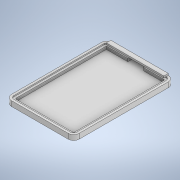
# Autodesk Inventor part: piholder-v1
Saved by Autodesk Inventor 2022 (Build 260153000, 153)
## iProperties
Created: 2021-07-08
Part Number: piholder-v1
Material: Generic
Document SubType Name: Modeling
Designer: dncob
Density: 1 g/cm^3
Appearance: Default
Author: dncob
Autodesk Inventor part; units mm, degrees
ref_plane "YZ Plane" through (0, 0, 0) normal (1, 0, 0) x (0, 1, 0)
ref_plane "XZ Plane" through (0, 0, 0) normal (0, 1, 0) x (-1, 0, 0)
ref_plane "XY Plane" through (0, 0, 0) normal (0, 0, 1) x (1, 0, 0)
sketch "Sketch1" plane through (0, 0, 0) normal (0, 1, 0) x (-1, 0, 0)
  line L0 (-25, 42.5) -> (25, 42.5)
  line L1 (28, 39.5) -> (28, -40.5)
  line L2 (26, -42.5) -> (-25, -42.5)
  line L3 (-28, -39.5) -> (-28, 39.5)
  line L4 (-28, 42.5) -> (28, -42.5) construction
  line L5 (28, 42.5) -> (-28, -42.5) construction
  arc A0 (26, -42.5) -> (28, -40.5) centre (26, -40.5) ccw
  arc A1 (-28, -39.5) -> (-25, -42.5) centre (-25, -39.5) ccw
  arc A2 (-25, 42.5) -> (-28, 39.5) centre (-25, 39.5) ccw
  arc A3 (28, 39.5) -> (25, 42.5) centre (25, 39.5) ccw
  line L6 (30, -40.5) -> (30, 39.5)
  arc A4 (30, 39.5) -> (25, 44.5) centre (25, 39.5) ccw
  line L7 (25, 44.5) -> (-25, 44.5)
  arc A5 (-25, 44.5) -> (-30, 39.5) centre (-25, 39.5) ccw
  line L8 (-30, 39.5) -> (-30, -39.5)
  arc A6 (-30, -39.5) -> (-25, -44.5) centre (-25, -39.5) ccw
  line L9 (-25, -44.5) -> (26, -44.5)
  arc A7 (26, -44.5) -> (30, -40.5) centre (26, -40.5) ccw
  point P0 (0, 0)
  dimension "d0" = 56
  dimension "d1" = 85
  dimension "d2" = 2
  dimension "d3" = 3
  dimension "d4" = 2
  constraints: 20 end point, 16 point on circle, 8 centre point, 8 point on line, 8 tangent, 4 parallel, 2 equal radius, 2 midpoint, 2 perpendicular, 1 horizontal, 7 other
  measures "d0" distance of L4.end L5.end
  measures "d1" distance of L5.start L4.end
  measures "d2" radius of A0
  measures "d3" radius of A1
  measures "d4" distance between parallel lines of L1 L6
extrude "Extrusion1" add sketch "Sketch1" along normal blind 1
sketch "Sketch2" plane through (0, 0, 0) normal (0, -1, 0) x (1, 0, 0)
  arc A0 (-25, 44.5) -> (-30, 39.5) centre (-25, 39.5) ccw projected
  line L0 (-25, 44.5) -> (25, 44.5) projected
  arc A1 (30, 39.5) -> (25, 44.5) centre (25, 39.5) ccw projected
  line L1 (30, 39.5) -> (30, -39.5) projected
  arc A2 (25, -44.5) -> (30, -39.5) centre (25, -39.5) ccw projected
  line L2 (25, -44.5) -> (-26, -44.5) projected
  arc A3 (-30, -40.5) -> (-26, -44.5) centre (-26, -40.5) ccw projected
  line L3 (-30, -40.5) -> (-30, 39.5) projected
  line L4 (-26, -44.5) -> (25, -44.5)
  line L5 (30, -39.5) -> (30, 39.5)
  line L6 (25, 44.5) -> (-25, 44.5)
  line L7 (-30, 39.5) -> (-30, -40.5)
  line L8 (-30, -44.5) -> (30, 44.5) construction
  line L9 (30, -44.5) -> (-30, 44.5) construction
  arc A4 (-25, 44.5) -> (-30, 39.5) centre (-25, 39.5) ccw
  arc A5 (30, 39.5) -> (25, 44.5) centre (25, 39.5) ccw
  arc A6 (25, -42.5) -> (28, -39.5) centre (25, -39.5) ccw projected
  arc A7 (25, -44.5) -> (30, -39.5) centre (25, -39.5) ccw
  arc A8 (-30, -40.5) -> (-26, -44.5) centre (-26, -40.5) ccw
  line L10 (25, 40.5) -> (-25, 40.5)
  arc A9 (-25, 40.5) -> (-26, 39.5) centre (-25, 39.5) ccw
  line L11 (-26, 39.5) -> (-26, -40.5)
  line L12 (-26, -40.5) -> (25, -40.5)
  arc A10 (25, -40.5) -> (26, -39.5) centre (25, -39.5) ccw
  line L13 (26, -39.5) -> (26, 39.5)
  arc A11 (26, 39.5) -> (25, 40.5) centre (25, 39.5) ccw
  point P0 (0, 0)
  point P1 (-26, -40.5)
  dimension "d12" = 4
  constraints: 21 end point, 14 point on circle, 7 centre point, 4 coincident, 4 concentric, 4 point on line, 2 collinear, 2 midpoint, 2 parallel, 1 horizontal, 1 perpendicular, 11 other
  measures "d12" distance between parallel lines of L10 L0
extrude "Extrusion2" add sketch "Sketch2" along normal blind 2.5
sketch "Sketch3" plane through (25, 1, -44.5) normal (0, 0, -1) x (-1, 0, 0)
  line L0 (51, -3.5) -> (51, 0) projected
  line L1 (51, 0) -> (0, 0)
  line L2 (0, 0) -> (0, 1.5)
  line L3 (0, 1.5) -> (51, 1.5)
  line L4 (51, 1.5) -> (51, 0)
  point P0 (25, -1)
  dimension "d9" = 1.5
  constraints: 8 end point, 2 parallel, 1 coincident, 1 horizontal, 1 perpendicular
  measures "d9" distance between parallel lines of L1 L3
extrude "Extrusion3" add sketch "Sketch3" against normal blind 4
sketch "Sketch4" plane through (0, -2.5, 0) normal (0, -1, 0) x (1, 0, 0)
  line L0 (25, 44.5) -> (-25, 44.5)
  line L1 (-30, 39.5) -> (-30, -40.5)
  line L2 (-26, -44.5) -> (25, -44.5)
  line L3 (30, -39.5) -> (30, 39.5)
  line L4 (30, 44.5) -> (-30, -44.5) construction
  line L5 (-30, 44.5) -> (30, -44.5) construction
  line L6 (-26, -44.5) -> (25, -44.5) projected
  line L7 (-30, 39.5) -> (-30, -40.5) projected
  arc A0 (25, -44.5) -> (30, -39.5) centre (25, -39.5) ccw projected
  arc A1 (-30, -40.5) -> (-26, -44.5) centre (-26, -40.5) ccw projected
  arc A2 (-25, 44.5) -> (-30, 39.5) centre (-25, 39.5) ccw projected
  arc A3 (30, 39.5) -> (25, 44.5) centre (25, 39.5) ccw projected
  arc A4 (25, -44.5) -> (30, -39.5) centre (25, -39.5) ccw
  line L8 (25, -40.5) -> (-26, -40.5) projected
  arc A5 (-30, -40.5) -> (-26, -44.5) centre (-26, -40.5) ccw
  arc A6 (-25, 44.5) -> (-30, 39.5) centre (-25, 39.5) ccw
  arc A7 (30, 39.5) -> (25, 44.5) centre (25, 39.5) ccw
  line L9 (25, 44.5) -> (-25, 44.5) projected
  point P0 (0, 0)
  constraints: 13 end point, 10 point on circle, 4 centre point, 4 coincident, 4 concentric, 4 point on line, 3 collinear, 2 midpoint, 2 parallel, 1 horizontal, 1 perpendicular
extrude "Extrusion4" add sketch "Sketch4" along normal blind 1
sketch "Sketch5" plane through (25, 2.5, -44.5) normal (0, 0, -1) x (-1, 0, 0)
  line L0 (51, -6) -> (0, -6) projected
  line L1 (18, -5) -> (32, -5)
  line L2 (32, -5) -> (32, -2.5)
  line L3 (32, -2.5) -> (18, -2.5)
  line L4 (18, -2.5) -> (18, -5)
  line L5 (18, -5) -> (32, -2.5) construction
  line L6 (32, -5) -> (18, -2.5) construction
  point P0 (25, -2.5)
  point P1 (25, -3.75)
  dimension "d16" = 14
  dimension "d17" = 1
  dimension "d18" = 2.5
  constraints: 12 end point, 2 midpoint, 2 parallel, 1 horizontal, 1 perpendicular, 1 vertical alignment
  measures "d16" distance of L2.end L3.end
  measures "d17" distance between parallel lines of L0 L1
  measures "d18" distance between parallel lines of L1 L3
extrude "Extrusion5" cut sketch "Sketch5" against normal up to surface (4 mm away)
body "Solid1"
